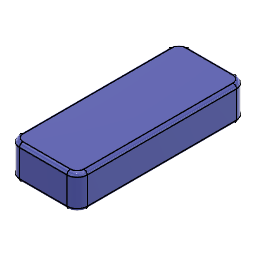
Case (Autodesk Fusion 360 archive; units mm, degrees)
design "Cantor Battery"
Autodesk Fusion 360 part; units mm, degrees
sketch "Sketch1" plane through (0, 0, 0) normal (0, 1, 0) x (1, 0, 0)
  line L0 (0, 0) -> (20, 0)
  line L1 (20, 0) -> (20, -50)
  line L2 (20, -50) -> (0, -50)
  line L3 (0, -50) -> (0, 0)
  dimension "d1" = 20
  dimension "d2" = 50
  constraint horizontal L0
  constraint vertical L1
  constraint horizontal L2
  constraint vertical L3
  constraint coincident L0.start L3.end
  measures "d1" distance of L0.start L0.end
  measures "d2" distance of L0.start L2.end
extrude "Extrude1" add sketch "Sketch1" along normal blind 10
fillet "Fillet1" radius 3 4 edges at (20, 5, 50) (0, 5, 50) (0, 5, 0) (20, 5, 0)
fillet "Fillet1" radius 1 2 faces at (6.6667, 10, 16.6667) (6.6667, 0, 16.6667)
